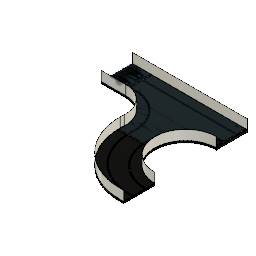
_1-5 (Entrance).d2b125fc-16cf-42d4-bfd9-f85618610363 (Autodesk Fusion 360 design; units mm, degrees)
Autodesk Fusion 360 part; units mm, degrees
note: some values were not read from the file. Chosen so that the rebuilt part matches the saved one: which bodies a step acts on. Set by a fixed rule: which sketch regions a step uses.
sketch "Sketch1" plane through (0, 0, 0) normal (0, 0, 1) x (1, 0, 0)
  line L0 (0, 0) -> (609.6, 0)
  line L1 (609.6, -812.8) -> (0, -812.8)
  line L2 (0, -812.8) -> (0, 0)
  line L3 (0, 0) -> (3022.6, 0)
  line L4 (3022.6, 0) -> (0, 0)
  line L5 (0, 0) -> (0, -812.8)
  line L6 (0, -812.8) -> (3022.6, -812.8)
  line L7 (0, 0) -> (1320.8, 0)
  circle A0 centre (4656.6619, -4772.6092) radius 793.75
  circle A1 centre (4656.6619, -4772.6092) radius 1625.6
  circle A2 centre (2997.2, -1612.9) radius 1612.9
  circle A3 centre (2997.2, -1612.9) radius 800.1
  line L8 (2997.2, -1612.9) -> (2997.2, 0)
  line L9 (2997.2, -1612.9) -> (2997.2, -3225.8)
  line L10 (3022.6, 0) -> (2997.2, 0)
  line L11 (2997.2, 0) -> (2997.2, -812.8)
  line L12 (2997.2, -812.8) -> (3022.6, -812.8)
  line L13 (2997.2, -1612.9) -> (1295.4, -1612.9)
  arc A4 (1384.3, -1612.9) -> (2997.2, -3225.8) centre (2997.2, -1612.9) ccw
  arc A5 (1384.3, -1612.9) -> (2997.2, -3225.8) centre (2997.2, -1612.9) ccw
  line L14 (2997.2, -1612.9) -> (1806.0752, -2792.535)
  arc A6 (1295.4, -1612.9) -> (2997.2, -3225.8) centre (2908.8371, -1614.7833) ccw
  arc A7 (2997.2, 0) -> (1295.4, -1612.9) centre (2908.8371, -1611.0167) ccw
  circle A8 centre (639.1793, -1473.2) radius 660.4
  dimension "d1" = 609.6
  dimension "d2" = 812.8
  dimension "d4" = 3022.6
  dimension "d8" = 1320.8
  dimension "d10" = 1587.5
  dimension "d11" = 3251.2
  dimension "d14" = 25.4
  dimension "d15" = 1701.8
  dimension "d16" = 1676.4
  dimension "d18" = 1320.8
  constraint horizontal L0
  constraint horizontal L1
  constraint vertical L2
  constraint coincident L0.start L2.end
  constraint perpendicular L2 L3
  constraint horizontal L4
  constraint vertical L5
  constraint horizontal L6
  constraint perpendicular L5 L7
  constraint concentric A0 A1
  constraint concentric A2 A3
  constraint coincident A2.centre A3.centre
  constraint coincident A2 L8.end
  constraint vertical L8
  constraint coincident A2 L9.end
  constraint parallel L8 L9
  constraint horizontal L10
  constraint vertical L11
  constraint horizontal L12
  constraint coincident L14.end A6
  constraint symmetric L9.end L13 L8.end
  constraint symmetric A6.start L13 A7.end
  constraint symmetric L13 A6 A7
  constraint tangent L6 A8
  constraint tangent A7 A8
  measures "d1" distance of L0.start L0.end
  measures "d2" distance of L0.start L1.end
  measures "d4" distance of L0.start L3.end
  measures "d8" distance of L0.start L7.end
  measures "d10" diameter of A0
  measures "d11" diameter of A1
  measures "d14" distance of L3.end L8.end
  measures "d15" distance of A2.centre L13.end
  measures "d16" distance of A2.centre L14.end
  measures "d18" diameter of A8
extrude "Extrude1" add sketch "Sketch1" along normal blind 50.8 contours L0 L1 L2 L3 L4 L5 L6 L7 A7 | L3 L4 L6 A2 A7 | L6 A7 A8 | L6 A2 L8 L11 | L6 A2 L13 A7 | L6 A2 A3 L13 | A2 L13 A4 A5 L14 A6 | A2 A4 A5 L14 A6 | A2 A3 L9 A4 A5 L14 | A2 A3 L13 A4 A5 L14 makes body 1
sketch "Lines" plane through (0, 0, 50.8) normal (0, 0, 1) x (-1, 0, 0)
  arc A0 (-1295.4, 1612.9) -> (-2997.2, 3225.8) centre (-2908.8371, 1614.7833) ccw
  line L0 (-2997.2, 3225.8) -> (-2997.2, 2413)
  arc A1 (-2997.2, 812.8) -> (-2997.2, 2413) centre (-2997.2, 1612.9) ccw
  line L1 (-2997.2, 812.8) -> (-2997.2, 0)
  line L2 (-2997.2, 0) -> (0, 0)
  line L3 (0, 0) -> (0, 812.8)
  line L4 (0, 812.8) -> (-639.1793, 812.8)
  arc A2 (-1298.3651, 1513.2267) -> (-639.1793, 812.8) centre (-639.1793, 1473.2) ccw
  arc A3 (-1298.3651, 1513.2267) -> (-1295.4, 1612.9) centre (-2908.8371, 1611.0167) ccw
  line L5 (0, 431.8) -> (-482.6, 431.8)
  line L6 (-482.6, 431.8) -> (-511.175, 431.8)
  line L7 (-511.175, 431.8) -> (-511.175, 812.8)
  line L8 (-511.175, 812.8) -> (-482.6, 812.8)
  line L9 (-482.6, 812.8) -> (-482.6, 431.8)
  line L10 (-511.175, 812.8) -> (-482.6, 812.8)
  line L11 (-482.6, 812.8) -> (-482.6, 0)
  line L12 (-482.6, 0) -> (-511.175, 0)
  line L13 (-511.175, 0) -> (-511.175, 812.8)
  line L14 (-1651, 0) -> (-1651, 1651)
  line L15 (-1651, 1651) -> (-1291.2162, 1651)
  line L16 (-1291.2162, 1651) -> (-1291.2162, 1679.575)
  line L17 (-1291.2162, 1679.575) -> (-1651, 1679.575)
  line L18 (-1651, 1679.575) -> (-1651, 1651)
  line L19 (-1291.2162, 1679.575) -> (-2198.0077, 1679.575)
  line L20 (-2198.0077, 1679.575) -> (-2198.0077, 1651)
  line L21 (-2198.0077, 1651) -> (-1291.2162, 1651)
  line L22 (-1291.2162, 1651) -> (-1291.2162, 1679.575)
  line L23 (0, 431.8) -> (-2946.4, 431.8)
  line L24 (-2946.4, 431.8) -> (-2974.975, 431.8)
  line L25 (-2974.975, 431.8) -> (-2974.975, 813.6871)
  line L26 (-2974.975, 813.6871) -> (-2946.4, 813.6871)
  line L27 (-2946.4, 813.6871) -> (-2946.4, 431.8)
  line L28 (-2974.975, 431.8) -> (-2946.4, 431.8)
  line L29 (-2946.4, 431.8) -> (-2946.4, 0)
  line L30 (-2946.4, 0) -> (-2974.975, 0)
  line L31 (-2974.975, 0) -> (-2974.975, 431.8)
  dimension "d45" = 482.6
  dimension "d46" = 28.575
  dimension "d47" = 1651
  dimension "d48" = 28.575
  dimension "d49" = 2946.4
  dimension "d50" = 28.575
  constraint coincident L3 L5.start
  constraint perpendicular L3 L5
  constraint horizontal L6
  constraint vertical L7
  constraint horizontal L8
  constraint vertical L9
  constraint horizontal L10
  constraint vertical L11
  constraint horizontal L12
  constraint vertical L13
  constraint coincident L2 L11.end
  constraint coincident L2 L14.start
  constraint perpendicular L2 L14
  constraint horizontal L15
  constraint vertical L16
  constraint horizontal L17
  constraint vertical L18
  constraint horizontal L19
  constraint vertical L20
  constraint horizontal L21
  constraint vertical L22
  constraint coincident A1 L20.end
  constraint perpendicular L11 L23
  constraint horizontal L24
  constraint vertical L25
  constraint horizontal L26
  constraint vertical L27
  constraint horizontal L28
  constraint vertical L29
  constraint horizontal L30
  constraint vertical L31
  constraint coincident L2 L29.end
  measures "d45" distance of L5.start L5.end
  measures "d46" distance of L5.end L6.end
  measures "d47" distance of L14.start L14.end
  measures "d48" distance of L14.end L17.end
  measures "d49" distance of L5.start L23.end
  measures "d50" distance of L23.end L24.end
extrude "Extrude6" add sketch "Lines" along normal blind 0.0254 contours A0 L15 L17 L18 L19 L21 | L18 L19 L20 L21 | L4 L6 L7 L8 L9 L10 L11 L13 L23 | L2 L6 L11 L12 L13 L23 | L2 L24 L28 L29 L30 L31 | A1 L24 L25 L26 L27 L28 bodies 1
sketch "Sketch7" plane through (0, 0, 50.8) normal (0, 0, 1) x (-1, 0, 0)
  line L0 (-2959.5333, 813.6871) -> (-2946.4, 813.6871)
  line L1 (-2946.4, 813.6871) -> (-2946.4, 0)
  line L2 (-2946.4, 0) -> (-511.175, 0)
  line L3 (-511.175, 0) -> (-511.175, 812.8)
  line L4 (-511.175, 812.8) -> (-639.1793, 812.8)
  arc A0 (-1298.3651, 1513.2267) -> (-639.1793, 812.8) centre (-639.1793, 1473.2) ccw
  arc A1 (-1298.3651, 1513.2267) -> (-1295.4, 1612.9) centre (-2908.8371, 1611.0167) ccw
  arc A2 (-1295.4, 1612.9) -> (-1295.8054, 1651) centre (-2908.8371, 1614.7833) ccw
  line L5 (-1295.8054, 1651) -> (-2198.0077, 1651)
  arc A3 (-2959.5333, 813.6871) -> (-2198.0077, 1651) centre (-2997.2, 1612.9) ccw
  line L6 (-482.6, 812.8) -> (-482.6, 0)
  line L7 (-482.6, 0) -> (0, 0)
  line L8 (0, 0) -> (0, 812.8)
  line L9 (0, 812.8) -> (-482.6, 812.8)
  line L10 (-2198.0077, 1679.575) -> (-1296.7004, 1679.575)
  arc A4 (-1296.7004, 1679.575) -> (-2997.2, 3225.8) centre (-2908.8371, 1614.7833) ccw
  line L11 (-2997.2, 3225.8) -> (-2997.2, 2413)
  arc A5 (-2198.0077, 1651) -> (-2997.2, 2413) centre (-2997.2, 1612.9) ccw
  line L12 (-2198.0077, 1651) -> (-2198.0077, 1679.575)
  line L13 (-2997.2, 812.8) -> (-2997.2, 0)
  line L14 (-574.675, 749.3) -> (-639.1793, 749.3)
  arc A6 (-1361.7484, 1517.0754) -> (-639.1793, 749.3) centre (-639.1793, 1473.2) ccw
  arc A7 (-1361.7484, 1517.0754) -> (-1359.0773, 1587.5) centre (-2908.8371, 1611.0167) ccw
  line L15 (-1359.0773, 1587.5) -> (-2133.9736, 1587.5)
  arc A8 (-2882.9, 756.8974) -> (-2133.9736, 1587.5) centre (-2997.2, 1612.9) ccw
  line L16 (-2882.9, 756.8974) -> (-2882.9, 63.5)
  line L17 (-2882.9, 63.5) -> (-574.675, 63.5)
  line L18 (-574.675, 63.5) -> (-574.675, 749.3)
  circle A9 centre (-793.75, 765.9949) radius 16
  circle A10 centre (-2171.7977, 1358.9) radius 16
  circle A11 centre (-1353.9986, 1358.9) radius 16
  circle A12 centre (-2768.6, 63.5) radius 16
  dimension "d53" = 63.5
  dimension "d55" = 32
  dimension "d59" = 32
  dimension "d60" = 32
  dimension "d62" = 32
  measures "d55" diameter of A9
  measures "d59" diameter of A10
  measures "d60" diameter of A11
  measures "d62" diameter of A12
extrude "Extrude7" add sketch "Sketch7" along normal blind 0.0254 contours A6 A9 | A6 A9 | L17 A12 | L17 A12 | A6 A11 | A6 A11 | A8 A10 | A8 A10 bodies 1
sketch "Sketch8" plane through (0, 0, 50.8) normal (0, 0, 1) x (-1, 0, 0)
  line L0 (-482.6, 812.8) -> (-482.6, 0)
  line L1 (-482.6, 0) -> (0, 0)
  line L2 (0, 0) -> (0, 812.8)
  line L3 (0, 812.8) -> (-482.6, 812.8)
  line L4 (-482.6, 231.775) -> (0, 231.775)
  line L5 (-482.6, 250.825) -> (0, 250.825)
  line L6 (0, 561.975) -> (-482.6, 561.975)
  line L7 (0, 581.025) -> (-482.6, 581.025)
  dimension "d66" = -250.825
extrude "Extrude8" add sketch "Sketch8" along normal blind 0.0254 contours L0 L2 L6 L7 | L0 L2 L4 L5 bodies 1
sketch "Sketch9" plane through (0, 0, 50.8254) normal (0, 0, 1) x (-1, 0, 0)
  line L0 (-511.175, 0) -> (-482.6, 0)
  line L1 (-482.6, 0) -> (-482.6, 231.775)
  line L2 (-482.6, 231.775) -> (0, 231.775)
  line L3 (0, 231.775) -> (0, 250.825)
  line L4 (0, 250.825) -> (-482.6, 250.825)
  line L5 (-482.6, 250.825) -> (-482.6, 561.975)
  line L6 (-482.6, 561.975) -> (0, 561.975)
  line L7 (0, 561.975) -> (0, 581.025)
  line L8 (0, 581.025) -> (-482.6, 581.025)
  line L9 (-482.6, 581.025) -> (-482.6, 812.8)
  line L10 (-482.6, 812.8) -> (-511.175, 812.8)
  line L11 (-511.175, 812.8) -> (-511.175, 0)
  line L12 (-482.6, 231.775) -> (-482.5746, 231.775)
  line L13 (-482.5746, 231.775) -> (-482.5746, 250.825)
  line L14 (-482.5746, 250.825) -> (-482.6, 250.825)
  line L15 (-482.6, 250.825) -> (-482.6, 231.775)
  dimension "d71" = 0.0254
  constraint horizontal L12
  constraint vertical L13
  constraint horizontal L14
  constraint vertical L15
  constraint coincident L1.end L2.start
  measures "d71" distance of L1.end L12.end
extrude "Extrude9" cut sketch "Sketch9" against normal blind 0.0254 contours L2 L4 L12 L13 L14 L15 bodies 1
sketch "Sketch10" plane through (0, 0, 50.8) normal (0, 0, 1) x (-1, 0, 0)
  line L0 (-482.6, 581.025) -> (0, 581.025)
  line L1 (0, 581.025) -> (0, 812.8)
  line L2 (0, 812.8) -> (-482.6, 812.8)
  line L3 (-482.6, 812.8) -> (-482.6, 581.025)
sketch "Sketch11" plane through (0, 0, 50.8254) normal (0, 0, 1) x (-1, 0, 0)
  line L0 (-482.6, 0) -> (-482.6, 561.975)
  line L1 (-482.6, 561.975) -> (0, 561.975)
  line L2 (0, 561.975) -> (0, 581.025)
  line L3 (0, 581.025) -> (-482.6, 581.025)
  line L4 (-482.6, 581.025) -> (-482.6, 812.8)
  line L5 (-482.6, 812.8) -> (-511.175, 812.8)
  line L6 (-511.175, 812.8) -> (-511.175, 0)
  line L7 (-511.175, 0) -> (-482.6, 0)
  line L8 (-482.6, 561.975) -> (-482.5746, 561.975)
  line L9 (-482.5746, 561.975) -> (-482.5746, 581.025)
  line L10 (-482.5746, 581.025) -> (-482.6, 581.025)
  line L11 (-482.6, 581.025) -> (-482.6, 561.975)
  dimension "d74" = 0.0254
  constraint horizontal L8
  constraint vertical L9
  constraint horizontal L10
  constraint vertical L11
  constraint coincident L0.end L1.start
  measures "d74" distance of L0.end L8.end
extrude "Extrude10" cut sketch "Sketch11" against normal blind 0.0254 contours L1 L3 L8 L9 L10 L11 bodies 1
sketch "Sketch12" plane through (0, 0, 50.8) normal (0, 0, 1) x (-1, 0, 0)
  circle A0 centre (-2768.6, 63.5) radius 16
  circle A1 centre (-793.75, 765.9949) radius 16
  circle A2 centre (-2171.7977, 1358.9) radius 16
  circle A3 centre (-1353.9986, 1358.9) radius 16
  line L0 (-2959.5333, 813.6871) -> (-2946.4, 813.6871)
  line L1 (-2946.4, 813.6871) -> (-2946.4, 0)
  line L2 (-2946.4, 0) -> (-511.175, 0)
  line L3 (-511.175, 0) -> (-511.175, 812.8)
  line L4 (-511.175, 812.8) -> (-639.1793, 812.8)
  arc A4 (-1298.3651, 1513.2267) -> (-639.1793, 812.8) centre (-639.1793, 1473.2) ccw
  arc A5 (-1298.3651, 1513.2267) -> (-1295.4, 1612.9) centre (-2908.8371, 1611.0167) ccw
  arc A6 (-1295.4, 1612.9) -> (-1295.8054, 1651) centre (-2908.8371, 1614.7833) ccw
  line L5 (-1295.8054, 1651) -> (-2198.0077, 1651)
  arc A7 (-2959.5333, 813.6871) -> (-2198.0077, 1651) centre (-2997.2, 1612.9) ccw
  line L6 (-2946.4, 250.825) -> (-511.175, 250.825)
  line L7 (-2946.4, 231.775) -> (-511.175, 231.775)
  dimension "d78" = -231.775
extrude "Extrude11" add sketch "Sketch12" along normal blind 0.0254 contours L1 L3 L6 L7 bodies 1
sketch "Sketch13" plane through (0, 0, 50.8254) normal (0, 0, 1) x (-1, 0, 0)
  line L0 (-482.6, 0) -> (-482.6, 812.8)
  line L1 (-482.6, 812.8) -> (-511.175, 812.8)
  line L2 (-511.175, 812.8) -> (-511.175, 250.825)
  line L3 (-511.175, 250.825) -> (-2946.4, 250.825)
  line L4 (-2946.4, 250.825) -> (-2946.4, 813.6871)
  line L5 (-2946.4, 813.6871) -> (-2959.5333, 813.6871)
  arc A0 (-2974.975, 813.1087) -> (-2959.5333, 813.6871) centre (-2997.2, 1612.9) ccw
  line L6 (-2974.975, 813.1087) -> (-2974.975, 0)
  line L7 (-2974.975, 0) -> (-2946.4, 0)
  line L8 (-2946.4, 0) -> (-2946.4, 231.775)
  line L9 (-2946.4, 231.775) -> (-511.175, 231.775)
  line L10 (-511.175, 231.775) -> (-511.175, 0)
  line L11 (-511.175, 0) -> (-482.6, 0)
  line L12 (-511.175, 250.825) -> (-511.2004, 250.825)
  line L13 (-511.2004, 250.825) -> (-511.2004, 231.775)
  line L14 (-511.2004, 231.775) -> (-511.175, 231.775)
  line L15 (-511.175, 231.775) -> (-511.175, 250.825)
  dimension "d81" = 0.0254
  constraint horizontal L12
  constraint vertical L13
  constraint horizontal L14
  constraint vertical L15
  constraint coincident L2.end L3.start
  measures "d81" distance of L2.end L12.end
extrude "Extrude12" cut sketch "Sketch13" against normal blind 0.0254 contours L3 L9 L12 L13 L14 L15 bodies 1
sketch "Sketch14" plane through (0, 0, 50.8254) normal (0, 0, 1) x (-1, 0, 0)
  line L0 (-511.2004, 231.775) -> (-511.2004, 250.825)
  line L1 (-511.2004, 250.825) -> (-2946.4, 250.825)
  line L2 (-2946.4, 250.825) -> (-2946.4, 813.6871)
  line L3 (-2946.4, 813.6871) -> (-2959.5333, 813.6871)
  arc A0 (-2974.975, 813.1087) -> (-2959.5333, 813.6871) centre (-2997.2, 1612.9) ccw
  line L4 (-2974.975, 813.1087) -> (-2974.975, 0)
  line L5 (-2974.975, 0) -> (-2946.4, 0)
  line L6 (-2946.4, 0) -> (-2946.4, 231.775)
  line L7 (-2946.4, 231.775) -> (-511.2004, 231.775)
  line L8 (-2946.4, 250.825) -> (-2946.3746, 250.825)
  line L9 (-2946.3746, 250.825) -> (-2946.3746, 231.775)
  line L10 (-2946.3746, 231.775) -> (-2946.4, 231.775)
  line L11 (-2946.4, 231.775) -> (-2946.4, 250.825)
  dimension "d84" = 0.0254
  constraint horizontal L8
  constraint vertical L9
  constraint horizontal L10
  constraint vertical L11
  constraint coincident L1.end L2.start
  measures "d84" distance of L1.end L8.end
extrude "Extrude13" cut sketch "Sketch14" against normal blind 0.0254 contours L1 L7 L8 L9 L10 L11 bodies 1
sketch "Sketch15" plane through (0, 0, 50.8) normal (0, 0, 1) x (-1, 0, 0)
  line L0 (-2974.975, 0) -> (-2974.975, 813.1087)
  arc A0 (-2997.2, 812.8) -> (-2974.975, 813.1087) centre (-2997.2, 1612.9) ccw
  line L1 (-2997.2, 812.8) -> (-2997.2, 0)
  line L2 (-2997.2, 0) -> (-2974.975, 0)
  line L3 (-2997.2, 231.775) -> (-2974.975, 231.775)
  line L4 (-2997.2, 250.825) -> (-2974.975, 250.825)
extrude "Extrude14" add sketch "Sketch15" along normal blind 0.0254 contours L0 L1 L3 L4 bodies 1
sketch "Sketch16" plane through (0, 0, 50.8254) normal (0, 0, 1) x (-1, 0, 0)
  line L0 (-2946.4, 0) -> (-2946.4, 813.6871)
  line L1 (-2946.4, 813.6871) -> (-2959.5333, 813.6871)
  arc A0 (-2974.975, 813.1087) -> (-2959.5333, 813.6871) centre (-2997.2, 1612.9) ccw
  line L2 (-2974.975, 813.1087) -> (-2974.975, 250.825)
  line L3 (-2974.975, 250.825) -> (-2997.2, 250.825)
  line L4 (-2997.2, 250.825) -> (-2997.2, 231.775)
  line L5 (-2997.2, 231.775) -> (-2974.975, 231.775)
  line L6 (-2974.975, 231.775) -> (-2974.975, 0)
  line L7 (-2974.975, 0) -> (-2946.4, 0)
  line L8 (-2974.975, 231.775) -> (-2975.0004, 231.775)
  line L9 (-2975.0004, 231.775) -> (-2975.0004, 250.825)
  line L10 (-2975.0004, 250.825) -> (-2974.975, 250.825)
  line L11 (-2974.975, 250.825) -> (-2974.975, 231.775)
  dimension "d93" = 0.0254
  constraint horizontal L8
  constraint vertical L9
  constraint horizontal L10
  constraint vertical L11
  constraint coincident L5.end L6.start
  measures "d93" distance of L5.end L8.end
extrude "Extrude15" cut sketch "Sketch16" against normal blind 0.0254 contours L3 L5 L8 L9 L10 L11 bodies 1
sketch "Sketch17" plane through (0, 0, 50.8) normal (0, 0, 1) x (-1, 0, 0)
  line L0 (-2975.0004, 231.775) -> (-2997.2, 231.775)
  line L1 (-2997.2, 231.775) -> (-2997.2, 0)
  line L2 (-2997.2, 0) -> (-2974.975, 0)
  line L3 (-2974.975, 0) -> (-2974.975, 813.1087)
  arc A0 (-2997.2, 812.8) -> (-2974.975, 813.1087) centre (-2997.2, 1612.9) ccw
  line L4 (-2997.2, 812.8) -> (-2997.2, 250.825)
  line L5 (-2997.2, 250.825) -> (-2975.0004, 250.825)
  line L6 (-2975.0004, 250.825) -> (-2975.0004, 231.775)
sketch "Sketch18" plane through (0, 0, 50.8) normal (0, 0, 1) x (-1, 0, 0)
  line L0 (-2946.3746, 250.825) -> (-511.2004, 250.825)
  line L1 (-511.2004, 250.825) -> (-511.2004, 231.775)
  line L2 (-511.2004, 231.775) -> (-2946.3746, 231.775)
  line L3 (-2946.3746, 231.775) -> (-2946.3746, 250.825)
  circle A0 centre (-2768.6, 63.5) radius 16
  line L4 (-2946.4, 813.6871) -> (-2946.4, 0)
  line L5 (-2946.4, 0) -> (-511.175, 0)
  line L6 (-511.175, 0) -> (-511.175, 812.8)
  line L7 (-511.175, 812.8) -> (-639.1793, 812.8)
  arc A1 (-1298.3651, 1513.2267) -> (-639.1793, 812.8) centre (-639.1793, 1473.2) ccw
  arc A2 (-1298.3651, 1513.2267) -> (-1295.4, 1612.9) centre (-2908.8371, 1611.0167) ccw
  arc A3 (-1295.4, 1612.9) -> (-1295.8054, 1651) centre (-2908.8371, 1614.7833) ccw
  line L8 (-1295.8054, 1651) -> (-2198.0077, 1651)
  arc A4 (-2959.5333, 813.6871) -> (-2198.0077, 1651) centre (-2997.2, 1612.9) ccw
  line L9 (-2959.5333, 813.6871) -> (-2946.4, 813.6871)
  circle A5 centre (-793.75, 765.9949) radius 16
  circle A6 centre (-2171.7977, 1358.9) radius 16
  circle A7 centre (-1353.9986, 1358.9) radius 16
  arc A8 (-1548.729, 1528.4291) -> (-639.1793, 561.975) centre (-639.1793, 1473.2) ccw
  line L10 (-511.175, 561.975) -> (-639.1793, 561.975)
  arc A9 (-1529.714, 1527.2745) -> (-639.1793, 581.025) centre (-639.1793, 1473.2) ccw
  line L11 (-511.175, 581.025) -> (-639.1793, 581.025)
  arc A10 (-1529.714, 1527.2745) -> (-1527.1752, 1612.9) centre (-2908.8371, 1611.0167) ccw
  arc A11 (-1527.1752, 1612.9) -> (-1527.522, 1645.7974) centre (-2908.8371, 1614.7833) ccw
  arc A12 (-1548.729, 1528.4291) -> (-1546.2252, 1612.9) centre (-2908.8371, 1611.0167) ccw
  arc A13 (-1546.2252, 1612.9) -> (-1546.5672, 1645.3698) centre (-2908.8371, 1614.7833) ccw
  line L12 (-1527.522, 1645.7974) -> (-1527.522, 1651)
  line L13 (-1546.5672, 1645.3698) -> (-1546.5672, 1651)
  line L14 (-1527.522, 1651) -> (-1546.5672, 1651)
  dimension "d96" = -250.825
  dimension "d97" = -231.775
  dimension "d99" = -250.825
  constraint vertical L12
  constraint coincident L8 L12.end
  constraint vertical L13
  constraint coincident L8 L13.end
extrude "Extrude16" add sketch "Sketch18" along normal blind 0.0254 contours L6 L8 A8 L10 A9 L11 A10 A11 A12 A13 L12 L13 L14 bodies 1
sketch "Sketch19" plane through (0, 0, 50.8254) normal (0, 0, 1) x (-1, 0, 0)
  line L0 (-2198.0077, 1651) -> (-1546.5672, 1651)
  line L1 (-1546.5672, 1651) -> (-1546.5672, 1645.3698)
  arc A0 (-1546.2252, 1612.9) -> (-1546.5672, 1645.3698) centre (-2908.8371, 1614.7833) ccw
  arc A1 (-1548.729, 1528.4291) -> (-1546.2252, 1612.9) centre (-2908.8371, 1611.0167) ccw
  arc A2 (-1548.729, 1528.4291) -> (-639.1793, 561.975) centre (-639.1793, 1473.2) ccw
  line L2 (-639.1793, 561.975) -> (-511.175, 561.975)
  line L3 (-511.175, 561.975) -> (-511.175, 0)
  line L4 (-511.175, 0) -> (-482.6, 0)
  line L5 (-482.6, 0) -> (-482.6, 812.8)
  line L6 (-482.6, 812.8) -> (-511.175, 812.8)
  line L7 (-511.175, 812.8) -> (-511.175, 581.025)
  line L8 (-511.175, 581.025) -> (-639.1793, 581.025)
  arc A3 (-1529.714, 1527.2745) -> (-639.1793, 581.025) centre (-639.1793, 1473.2) ccw
  arc A4 (-1529.714, 1527.2745) -> (-1527.1752, 1612.9) centre (-2908.8371, 1611.0167) ccw
  arc A5 (-1527.1752, 1612.9) -> (-1527.522, 1645.7974) centre (-2908.8371, 1614.7833) ccw
  line L9 (-1527.522, 1645.7974) -> (-1527.522, 1651)
  line L10 (-1527.522, 1651) -> (-1295.8054, 1651)
  arc A6 (-1295.8054, 1651) -> (-1296.7004, 1679.575) centre (-2908.8371, 1614.7833) ccw
  line L11 (-1296.7004, 1679.575) -> (-2198.0077, 1679.575)
  line L12 (-2198.0077, 1679.575) -> (-2198.0077, 1651)
  line L13 (-511.175, 561.975) -> (-511.2004, 561.975)
  line L14 (-511.2004, 561.975) -> (-511.2004, 581.025)
  line L15 (-511.2004, 581.025) -> (-511.175, 581.025)
  line L16 (-511.175, 581.025) -> (-511.175, 561.975)
  dimension "d102" = 0.0254
  constraint horizontal L13
  constraint vertical L14
  constraint horizontal L15
  constraint vertical L16
  constraint coincident L2.end L3.start
  measures "d102" distance of L2.end L13.end
extrude "Extrude17" cut sketch "Sketch19" against normal blind 0.0254 contours L2 L8 L13 L14 L15 L16 bodies 1
sketch "Sketch20" plane through (0, 0, 50.8254) normal (0, 0, 1) x (-1, 0, 0)
  line L0 (-511.2004, 561.975) -> (-511.2004, 581.025)
  line L1 (-511.2004, 581.025) -> (-639.1793, 581.025)
  arc A0 (-1529.714, 1527.2745) -> (-639.1793, 581.025) centre (-639.1793, 1473.2) ccw
  arc A1 (-1529.714, 1527.2745) -> (-1527.1752, 1612.9) centre (-2908.8371, 1611.0167) ccw
  arc A2 (-1527.1752, 1612.9) -> (-1527.522, 1645.7974) centre (-2908.8371, 1614.7833) ccw
  line L2 (-1527.522, 1645.7974) -> (-1527.522, 1651)
  line L3 (-1527.522, 1651) -> (-1295.8054, 1651)
  arc A3 (-1295.8054, 1651) -> (-1296.7004, 1679.575) centre (-2908.8371, 1614.7833) ccw
  line L4 (-1296.7004, 1679.575) -> (-2198.0077, 1679.575)
  line L5 (-2198.0077, 1679.575) -> (-2198.0077, 1651)
  line L6 (-2198.0077, 1651) -> (-1546.5672, 1651)
  line L7 (-1546.5672, 1651) -> (-1546.5672, 1645.3698)
  arc A4 (-1546.2252, 1612.9) -> (-1546.5672, 1645.3698) centre (-2908.8371, 1614.7833) ccw
  arc A5 (-1548.729, 1528.4291) -> (-1546.2252, 1612.9) centre (-2908.8371, 1611.0167) ccw
  arc A6 (-1548.729, 1528.4291) -> (-639.1793, 561.975) centre (-639.1793, 1473.2) ccw
  line L8 (-639.1793, 561.975) -> (-511.2004, 561.975)
  line L9 (-1527.522, 1651) -> (-1546.5672, 1651)
  line L10 (-1546.5672, 1651) -> (-1546.5672, 1650.9746)
  line L11 (-1546.5672, 1650.9746) -> (-1527.522, 1650.9746)
  line L12 (-1527.522, 1650.9746) -> (-1527.522, 1651)
  dimension "d105" = 0.0254
  constraint horizontal L9
  constraint vertical L10
  constraint horizontal L11
  constraint vertical L12
  constraint coincident L2.end L3.start
  measures "d105" distance of L2.end L11.end
extrude "Extrude18" cut sketch "Sketch20" against normal blind 0.0254 contours L2 L7 L9 L10 L11 L12 bodies 1
sketch "Sketch21" plane through (0, 0, 50.8) normal (0, 0, 1) x (-1, 0, 0)
  line L0 (-1527.522, 1650.9746) -> (-1527.522, 1645.7974)
  arc A0 (-1527.1752, 1612.9) -> (-1527.522, 1645.7974) centre (-2908.8371, 1614.7833) ccw
  arc A1 (-1529.714, 1527.2745) -> (-1527.1752, 1612.9) centre (-2908.8371, 1611.0167) ccw
  arc A2 (-1529.714, 1527.2745) -> (-639.1793, 581.025) centre (-639.1793, 1473.2) ccw
  line L1 (-639.1793, 581.025) -> (-511.2004, 581.025)
  line L2 (-511.2004, 581.025) -> (-511.2004, 561.975)
  line L3 (-511.2004, 561.975) -> (-639.1793, 561.975)
  arc A3 (-1548.729, 1528.4291) -> (-639.1793, 561.975) centre (-639.1793, 1473.2) ccw
  arc A4 (-1548.729, 1528.4291) -> (-1546.2252, 1612.9) centre (-2908.8371, 1611.0167) ccw
  arc A5 (-1546.2252, 1612.9) -> (-1546.5672, 1645.3698) centre (-2908.8371, 1614.7833) ccw
  line L4 (-1546.5672, 1645.3698) -> (-1546.5672, 1650.9746)
  line L5 (-1546.5672, 1650.9746) -> (-1527.522, 1650.9746)
  circle A6 centre (-1353.9986, 1358.9) radius 16
  circle A7 centre (-793.75, 765.9949) radius 16
  line L6 (-1295.8054, 1651) -> (-2198.0077, 1651)
  arc A8 (-2959.5333, 813.6871) -> (-2198.0077, 1651) centre (-2997.2, 1612.9) ccw
  line L7 (-2959.5333, 813.6871) -> (-2946.4, 813.6871)
  line L8 (-2946.4, 813.6871) -> (-2946.4, 0)
  line L9 (-2946.4, 0) -> (-511.175, 0)
  line L10 (-511.175, 0) -> (-511.175, 812.8)
  line L11 (-511.175, 812.8) -> (-639.1793, 812.8)
  arc A9 (-1298.3651, 1513.2267) -> (-639.1793, 812.8) centre (-639.1793, 1473.2) ccw
  arc A10 (-1298.3651, 1513.2267) -> (-1295.4, 1612.9) centre (-2908.8371, 1611.0167) ccw
  arc A11 (-1295.4, 1612.9) -> (-1295.8054, 1651) centre (-2908.8371, 1614.7833) ccw
  line L12 (-2946.3746, 250.825) -> (-511.2004, 250.825)
  line L13 (-511.2004, 250.825) -> (-511.2004, 231.775)
  line L14 (-511.2004, 231.775) -> (-2946.3746, 231.775)
  line L15 (-2946.3746, 231.775) -> (-2946.3746, 250.825)
  circle A12 centre (-2768.6, 63.5) radius 16
  circle A13 centre (-2171.7977, 1358.9) radius 16
  arc A14 (-2947.7252, 563.1402) -> (-1947.4672, 1662.944) centre (-2997.2, 1612.9) ccw
  arc A15 (-2948.622, 582.1691) -> (-1966.4956, 1662.0369) centre (-2997.2, 1612.9) ccw
  dimension "d108" = 250.825
  dimension "d109" = 231.775
extrude "Extrude19" add sketch "Sketch21" along normal blind 0.0279 contours L6 L8 A14 A15 bodies 1
sketch "Sketch22" plane through (0, 0, 50.8) normal (0, 0, 1) x (-1, 0, 0)
sketch "Sketch23" plane through (0, 0, 50.8) normal (0, 0, 1) x (-1, 0, 0)
  line L0 (-1527.522, 1650.9746) -> (-1527.522, 1645.7974)
  arc A0 (-1527.1752, 1612.9) -> (-1527.522, 1645.7974) centre (-2908.8371, 1614.7833) ccw
  arc A1 (-1529.714, 1527.2745) -> (-1527.1752, 1612.9) centre (-2908.8371, 1611.0167) ccw
  arc A2 (-1529.714, 1527.2745) -> (-639.1793, 581.025) centre (-639.1793, 1473.2) ccw
  line L1 (-639.1793, 581.025) -> (-511.2004, 581.025)
  line L2 (-511.2004, 581.025) -> (-511.2004, 561.975)
  line L3 (-511.2004, 561.975) -> (-639.1793, 561.975)
  arc A3 (-1548.729, 1528.4291) -> (-639.1793, 561.975) centre (-639.1793, 1473.2) ccw
  arc A4 (-1548.729, 1528.4291) -> (-1546.2252, 1612.9) centre (-2908.8371, 1611.0167) ccw
  arc A5 (-1546.2252, 1612.9) -> (-1546.5672, 1645.3698) centre (-2908.8371, 1614.7833) ccw
  line L4 (-1546.5672, 1645.3698) -> (-1546.5672, 1650.9746)
  line L5 (-1546.5672, 1650.9746) -> (-1527.522, 1650.9746)
  circle A6 centre (-1353.9986, 1358.9) radius 16
  circle A7 centre (-793.75, 765.9949) radius 16
  arc A8 (-2946.4, 563.2035) -> (-1946.9659, 1651) centre (-2997.2, 1612.9) ccw
  line L6 (-2946.4, 563.2035) -> (-2946.4, 0)
  line L7 (-2946.4, 0) -> (-511.175, 0)
  line L8 (-511.175, 0) -> (-511.175, 812.8)
  line L9 (-511.175, 812.8) -> (-639.1793, 812.8)
  arc A9 (-1298.3651, 1513.2267) -> (-639.1793, 812.8) centre (-639.1793, 1473.2) ccw
  arc A10 (-1298.3651, 1513.2267) -> (-1295.4, 1612.9) centre (-2908.8371, 1611.0167) ccw
  arc A11 (-1295.4, 1612.9) -> (-1295.8054, 1651) centre (-2908.8371, 1614.7833) ccw
  line L10 (-1295.8054, 1651) -> (-1946.9659, 1651)
  line L11 (-2946.3746, 250.825) -> (-511.2004, 250.825)
  line L12 (-511.2004, 250.825) -> (-511.2004, 231.775)
  line L13 (-511.2004, 231.775) -> (-2946.3746, 231.775)
  line L14 (-2946.3746, 231.775) -> (-2946.3746, 250.825)
  circle A12 centre (-2768.6, 63.5) radius 16
sketch "Sketch24" plane through (0, 0, 50.8) normal (0, 0, 1) x (-1, 0, 0)
  line L0 (-2997.2, 812.8) -> (-2997.2, 581.025)
  line L1 (-2997.2, 812.8) -> (-2997.2, 561.975)
  line L2 (-2997.2, 561.975) -> (-2974.975, 561.975)
  line L3 (-2974.975, 561.975) -> (-2974.975, 581.025)
  line L4 (-2974.975, 581.025) -> (-2997.2, 581.025)
  line L5 (-2997.2, 581.025) -> (-2997.2, 561.975)
  line L6 (-2974.975, 0) -> (-2974.975, 813.1087)
  point P0 (-2997.2, 812.8)
  dimension "d112" = 231.775
  dimension "d113" = 250.825
  constraint coincident P0 L0.start
  constraint parallel L0 L1
  constraint horizontal L2
  constraint vertical L3
  constraint horizontal L4
  constraint vertical L5
  constraint coincident L3.end L6
  measures "d112" distance of P0 L0.end
  measures "d113" distance of P0 L1.end
extrude "Extrude20" add sketch "Sketch24" along normal blind 0.0279 bodies 1
extrude "Extrude21" cut sketch "Sketch24" along normal blind 0.0279 bodies 1
extrude "Extrude22" add sketch "Sketch24" along normal blind 0.0279 bodies 1
sketch "Sketch25" plane through (0, 0, 50.8) normal (0, 0, 1) x (-1, 0, 0)
  line L0 (-2198.0077, 1679.575) -> (-1296.7004, 1679.575)
  arc A0 (-1296.7004, 1679.575) -> (-2997.2, 3225.8) centre (-2908.8371, 1614.7833) ccw
  line L1 (-2997.2, 3225.8) -> (-2997.2, 2413)
  arc A1 (-2198.0077, 1651) -> (-2997.2, 2413) centre (-2997.2, 1612.9) ccw
  line L2 (-2198.0077, 1651) -> (-2198.0077, 1679.575)
  arc A2 (-1966.4956, 1662.0369) -> (-2997.2, 2644.775) centre (-2997.2, 1612.9) ccw
  arc A3 (-1947.4672, 1662.944) -> (-2997.2, 2663.825) centre (-2997.2, 1612.9) ccw
  dimension "d121" = 250.825
extrude "Extrude23" add sketch "Sketch25" along normal blind 0.0279 contours L0 L1 A2 A3 bodies 1
sketch "Sketch28" plane through (0, 0, 50.8) normal (0, 0, 1) x (-1, 0, 0)
  arc A0 (-1948.3922, 1679.575) -> (-2997.2, 2663.825) centre (-2997.2, 1612.9) ccw
  line L0 (-1948.3922, 1679.575) -> (-1296.7004, 1679.575)
  arc A1 (-1296.7004, 1679.575) -> (-2997.2, 3225.8) centre (-2908.8371, 1614.7833) ccw
  line L1 (-2997.2, 3225.8) -> (-2997.2, 2663.825)
  arc A2 (-1547.323, 1669.5025) -> (-2983.4631, 2975.3514) centre (-2908.8371, 1614.7833) ccw
  arc A3 (-1528.2884, 1670.2675) -> (-2984.5064, 2994.3729) centre (-2908.8371, 1614.7833) ccw
  line L2 (-2983.4631, 2975.3514) -> (-2997.2, 2974.598)
  line L3 (-2984.5064, 2994.3729) -> (-2997.2, 2993.6766)
  dimension "d125" = -231.775
  constraint coincident L1 L2.end
  constraint tangent A2 L2
  constraint coincident L1 L3.end
  constraint tangent A3 L3
extrude "Extrude24" add sketch "Sketch28" along normal blind 0.0279 contours L0 L1 A2 A3 L2 L3 bodies 1
sketch "Sketch29" plane through (0, 0, 0) normal (0, 0, -1) x (1, 0, 0)
  arc A0 (2997.2, 3225.8) -> (1295.4, 1612.9) centre (2908.8371, 1614.7833) ccw
  arc A1 (1295.4, 1612.9) -> (1298.3651, 1513.2267) centre (2908.8371, 1611.0167) ccw
  arc A2 (639.1793, 812.8) -> (1298.3651, 1513.2267) centre (639.1793, 1473.2) ccw
  line L0 (639.1793, 812.8) -> (0, 812.8)
  line L1 (0, 812.8) -> (0, 0)
  line L2 (0, 0) -> (2997.2, 0)
  line L3 (2997.2, 0) -> (2997.2, 812.8)
  arc A3 (2997.2, 2413) -> (2997.2, 812.8) centre (2997.2, 1612.9) ccw
  line L4 (2997.2, 2413) -> (2997.2, 3225.8)
  arc A4 (1295.654, 1612.9) -> (1298.6187, 1513.2421) centre (2908.8371, 1611.0167) ccw
  arc A5 (639.1793, 812.546) -> (1298.6187, 1513.2421) centre (639.1793, 1473.2) ccw
  line L5 (639.1793, 812.546) -> (0.254, 812.546)
  line L6 (0.254, 812.546) -> (0.254, 0.254)
  line L7 (0.254, 0.254) -> (2996.946, 0.254)
  line L8 (2996.946, 0.254) -> (2996.946, 812.546)
  arc A6 (2996.946, 2413.254) -> (2996.946, 812.546) centre (2997.2, 1612.9) ccw
  line L9 (2996.946, 2413.254) -> (2996.946, 3225.5595)
  arc A7 (2996.946, 3225.5595) -> (1295.654, 1612.9) centre (2908.8371, 1614.7833) ccw
  dimension "d128" = 0.254
extrude "Extrude25" add sketch "Sketch29" along normal blind 254 separate body contours  makes body 2
move_body "Move1" bodies 2 to x (1, 0, 0) y (0, 1, 0) z (0, 0, 1) at (0, 0, 304.8)
sketch "Sketch30" plane through (0, 0, 304.8) normal (0, 0, 1) x (-1, 0, 0)
  line L0 (-2996.946, 2413.254) -> (-2996.946, 3225.5595)
  arc A0 (-1295.654, 1612.9) -> (-2996.946, 3225.5595) centre (-2908.8371, 1614.7833) ccw
  arc A1 (-1298.6187, 1513.2421) -> (-1295.654, 1612.9) centre (-2908.8371, 1611.0167) ccw
  arc A2 (-1298.6187, 1513.2421) -> (-639.1793, 812.546) centre (-639.1793, 1473.2) ccw
  line L1 (-639.1793, 812.546) -> (-0.254, 812.546)
  line L2 (-0.254, 812.546) -> (-0.254, 0.254)
  line L3 (-0.254, 0.254) -> (-2996.946, 0.254)
  line L4 (-2996.946, 0.254) -> (-2996.946, 812.546)
  arc A3 (-2996.946, 812.546) -> (-2996.946, 2413.254) centre (-2997.2, 1612.9) ccw
  line L5 (0, 812.8) -> (-639.1793, 812.8)
  arc A4 (-1298.3651, 1513.2267) -> (-639.1793, 812.8) centre (-639.1793, 1473.2) ccw
  arc A5 (-1298.3651, 1513.2267) -> (-1295.4, 1612.9) centre (-2908.8371, 1611.0167) ccw
  arc A6 (-1295.4, 1612.9) -> (-2997.2, 3225.8) centre (-2908.8371, 1614.7833) ccw
  line L6 (-2997.2, 3225.8) -> (-2997.2, 2413)
  arc A7 (-2997.2, 812.8) -> (-2997.2, 2413) centre (-2997.2, 1612.9) ccw
  line L7 (-2997.2, 812.8) -> (-2997.2, 0)
  line L8 (-2997.2, 0) -> (0, 0)
  line L9 (0, 0) -> (0, 812.8)
  line L10 (-0.254, 812.546) -> (0, 812.546)
  line L11 (-0.254, 0.254) -> (0, 0.254)
  constraint coincident L1.end L2.start
  constraint coincident L9 L10.end
  constraint perpendicular L9 L10
  constraint coincident L2.end L3.start
  constraint coincident L9 L11.end
  constraint perpendicular L9 L11
extrude "Extrude26" cut sketch "Sketch30" against normal blind 254 contours L2 L9 L10 L11 bodies 1 2
sketch "Sketch31" plane through (0, 0, 304.8) normal (0, 0, 1) x (-1, 0, 0)
  line L0 (0, 0.254) -> (-2996.946, 0.254)
  line L1 (-2996.946, 0.254) -> (-2996.946, 812.546)
  arc A0 (-2996.946, 812.546) -> (-2996.946, 2413.254) centre (-2997.2, 1612.9) ccw
  line L2 (-2996.946, 2413.254) -> (-2996.946, 3225.5595)
  arc A1 (-1295.654, 1612.9) -> (-2996.946, 3225.5595) centre (-2908.8371, 1614.7833) ccw
  arc A2 (-1298.6187, 1513.2421) -> (-1295.654, 1612.9) centre (-2908.8371, 1611.0167) ccw
  arc A3 (-1298.6187, 1513.2421) -> (-639.1793, 812.546) centre (-639.1793, 1473.2) ccw
  line L3 (-639.1793, 812.546) -> (0, 812.546)
  line L4 (0, 812.546) -> (0, 812.8)
  line L5 (0, 812.8) -> (-639.1793, 812.8)
  arc A4 (-1298.3651, 1513.2267) -> (-639.1793, 812.8) centre (-639.1793, 1473.2) ccw
  arc A5 (-1298.3651, 1513.2267) -> (-1295.4, 1612.9) centre (-2908.8371, 1611.0167) ccw
  arc A6 (-1295.4, 1612.9) -> (-2997.2, 3225.8) centre (-2908.8371, 1614.7833) ccw
  line L6 (-2997.2, 3225.8) -> (-2997.2, 2413)
  arc A7 (-2997.2, 812.8) -> (-2997.2, 2413) centre (-2997.2, 1612.9) ccw
  line L7 (-2997.2, 812.8) -> (-2997.2, 0)
  line L8 (-2997.2, 0) -> (0, 0)
  line L9 (0, 0) -> (0, 0.254)
sketch "Sketch32" plane through (0, 0, 304.8) normal (0, 0, 1) x (-1, 0, 0)
  line L0 (-2997.2, 3225.8) -> (-2997.2, 2413)
  line L1 (-2996.946, 3225.5595) -> (-2997.2, 3225.5595)
  point P0 (-2996.946, 3225.5595)
  constraint coincident P0 L1.start
  constraint coincident L0 L1.end
  constraint perpendicular L0 L1
sketch "Sketch33" plane through (0, 0, 304.8) normal (0, 0, 1) x (-1, 0, 0)
  line L0 (0, 0.254) -> (-2996.946, 0.254)
  line L1 (-2996.946, 0.254) -> (-2996.946, 812.546)
  arc A0 (-2996.946, 812.546) -> (-2996.946, 2413.254) centre (-2997.2, 1612.9) ccw
  line L2 (-2996.946, 2413.254) -> (-2996.946, 3225.5595)
  arc A1 (-1295.654, 1612.9) -> (-2996.946, 3225.5595) centre (-2908.8371, 1614.7833) ccw
  arc A2 (-1298.6187, 1513.2421) -> (-1295.654, 1612.9) centre (-2908.8371, 1611.0167) ccw
  arc A3 (-1298.6187, 1513.2421) -> (-639.1793, 812.546) centre (-639.1793, 1473.2) ccw
  line L3 (-639.1793, 812.546) -> (0, 812.546)
  line L4 (0, 812.546) -> (0, 812.8)
  line L5 (0, 812.8) -> (-639.1793, 812.8)
  arc A4 (-1298.3651, 1513.2267) -> (-639.1793, 812.8) centre (-639.1793, 1473.2) ccw
  arc A5 (-1298.3651, 1513.2267) -> (-1295.4, 1612.9) centre (-2908.8371, 1611.0167) ccw
  arc A6 (-1295.4, 1612.9) -> (-2997.2, 3225.8) centre (-2908.8371, 1614.7833) ccw
  line L6 (-2997.2, 3225.8) -> (-2997.2, 2413)
  arc A7 (-2997.2, 812.8) -> (-2997.2, 2413) centre (-2997.2, 1612.9) ccw
  line L7 (-2997.2, 812.8) -> (-2997.2, 0)
  line L8 (-2997.2, 0) -> (0, 0)
  line L9 (0, 0) -> (0, 0.254)
  line L10 (-2996.946, 3225.5595) -> (-2997.2, 3225.5595)
  line L11 (-2996.946, 2413.254) -> (-2997.2, 2413.254)
  constraint coincident L2.end A1.end
  constraint perpendicular L2 L10
  constraint coincident A0.end L2.start
  constraint coincident L6 L11.end
  constraint tangent A0 L11
extrude "Extrude27" cut sketch "Sketch33" against normal blind 254 contours L2 L6 L10 L11 bodies 1 2 makes body 3 at (1951.3332, -2913.386, 135.4667)
sketch "Sketch34" plane through (0, 0, 304.8) normal (0, 0, 1) x (-1, 0, 0)
  line L0 (-2996.946, 2413.254) -> (-2997.2, 2413.254)
  line L1 (-2997.2, 2413.254) -> (-2997.2, 2413)
  arc A0 (-2997.2, 812.8) -> (-2997.2, 2413) centre (-2997.2, 1612.9) ccw
  line L2 (-2997.2, 812.8) -> (-2997.2, 0)
  line L3 (-2997.2, 0) -> (0, 0)
  line L4 (0, 0) -> (0, 0.254)
  line L5 (0, 0.254) -> (-2996.946, 0.254)
  line L6 (-2996.946, 0.254) -> (-2996.946, 812.546)
  arc A1 (-2996.946, 812.546) -> (-2996.946, 2413.254) centre (-2997.2, 1612.9) ccw
  line L7 (-2996.946, 812.546) -> (-2997.2, 812.546)
  line L8 (-2996.946, 0.254) -> (-2997.2, 0.254)
  constraint coincident L6.end A1.start
  constraint coincident L2 L7.end
  constraint tangent A1 L7
  constraint coincident L5.end L6.start
  constraint coincident L2 L8.end
  constraint perpendicular L2 L8
extrude "Extrude28" cut sketch "Sketch34" against normal blind 254 contours L2 L6 L7 L8 bodies 1 2 makes body 4 at (2917.2738, -816.5469, 220.1333)
sketch "Sketch35" plane through (0, 0, 50.8) normal (0, 0, 1) x (-1, 0, 0)
  line L0 (-1527.522, 1650.9746) -> (-1527.522, 1645.7974)
  arc A0 (-1527.1752, 1612.9) -> (-1527.522, 1645.7974) centre (-2908.8371, 1614.7833) ccw
  arc A1 (-1529.714, 1527.2745) -> (-1527.1752, 1612.9) centre (-2908.8371, 1611.0167) ccw
  arc A2 (-1529.714, 1527.2745) -> (-639.1793, 581.025) centre (-639.1793, 1473.2) ccw
  line L1 (-639.1793, 581.025) -> (-511.2004, 581.025)
  line L2 (-511.2004, 581.025) -> (-511.2004, 561.975)
  line L3 (-511.2004, 561.975) -> (-639.1793, 561.975)
  arc A3 (-1548.729, 1528.4291) -> (-639.1793, 561.975) centre (-639.1793, 1473.2) ccw
  arc A4 (-1548.729, 1528.4291) -> (-1546.2252, 1612.9) centre (-2908.8371, 1611.0167) ccw
  arc A5 (-1546.2252, 1612.9) -> (-1546.5672, 1645.3698) centre (-2908.8371, 1614.7833) ccw
  line L4 (-1546.5672, 1645.3698) -> (-1546.5672, 1650.9746)
  line L5 (-1546.5672, 1650.9746) -> (-1527.522, 1650.9746)
  circle A6 centre (-1353.9986, 1358.9) radius 16
  circle A7 centre (-793.75, 765.9949) radius 16
  arc A8 (-2946.4, 563.2035) -> (-1946.9659, 1651) centre (-2997.2, 1612.9) ccw
  line L6 (-2946.4, 563.2035) -> (-2946.4, 0)
  line L7 (-2946.4, 0) -> (-511.175, 0)
  line L8 (-511.175, 0) -> (-511.175, 812.8)
  line L9 (-511.175, 812.8) -> (-639.1793, 812.8)
  arc A9 (-1298.3651, 1513.2267) -> (-639.1793, 812.8) centre (-639.1793, 1473.2) ccw
  arc A10 (-1298.3651, 1513.2267) -> (-1295.4, 1612.9) centre (-2908.8371, 1611.0167) ccw
  arc A11 (-1295.4, 1612.9) -> (-1295.8054, 1651) centre (-2908.8371, 1614.7833) ccw
  line L10 (-1295.8054, 1651) -> (-1946.9659, 1651)
  line L11 (-2946.3746, 250.825) -> (-511.2004, 250.825)
  line L12 (-511.2004, 250.825) -> (-511.2004, 231.775)
  line L13 (-511.2004, 231.775) -> (-2946.3746, 231.775)
  line L14 (-2946.3746, 231.775) -> (-2946.3746, 250.825)
  circle A12 centre (-2768.6, 63.5) radius 16
sketch "Sketch36" plane through (0, 0, 50.8) normal (0, 0, 1) x (-1, 0, 0)
  line L0 (0, 0) -> (0, 812.8)
  line L1 (0, 812.8) -> (-482.6, 812.8)
  line L2 (-482.6, 812.8) -> (-482.6, 0)
  line L3 (-482.6, 0) -> (0, 0)
  line L4 (-0.254, 581.025) -> (-0.254, 561.975)
  line L5 (-0.254, 561.975) -> (-482.5746, 561.975)
  line L6 (-482.5746, 561.975) -> (-482.5746, 581.025)
  line L7 (-482.5746, 581.025) -> (-0.254, 581.025)
  line L8 (-0.254, 250.825) -> (-0.254, 231.775)
  line L9 (-0.254, 231.775) -> (-482.5746, 231.775)
  line L10 (-482.5746, 231.775) -> (-482.5746, 250.825)
  line L11 (-482.5746, 250.825) -> (-0.254, 250.825)
  line L12 (-0.254, 571.5) -> (-241.4143, 571.5)
  line L13 (-419.2143, 469.9) -> (-63.6143, 469.9)
  line L14 (-63.6143, 469.9) -> (-63.6143, 673.1)
  line L15 (-63.6143, 673.1) -> (-419.2143, 673.1)
  line L16 (-419.2143, 673.1) -> (-419.2143, 469.9)
  line L17 (-419.2143, 469.9) -> (-63.6143, 673.1) construction
  line L18 (-63.6143, 469.9) -> (-419.2143, 673.1) construction
  line L19 (-50.9143, 685.8) -> (-431.9143, 685.8)
  line L20 (-431.9143, 685.8) -> (-431.9143, 457.2)
  line L21 (-431.9143, 457.2) -> (-50.9143, 457.2)
  line L22 (-50.9143, 457.2) -> (-50.9143, 685.8)
  point P0 (-241.4143, 571.5)
  dimension "d140" = 241.1603
  dimension "d141" = 355.6
  dimension "d142" = 203.2
  dimension "d143" = 12.7
  constraint midpoint L4 L12.start
  constraint perpendicular L6 L12
  constraint horizontal L13
  constraint perpendicular L13 L14
  constraint parallel L13 L15
  constraint parallel L14 L16
  constraint coincident L17 P0
  constraint coincident L18 P0
  constraint coincident P0 L12.end
  measures "d140" distance of L12.start P0
  measures "d141" distance of L14.end L15.end
  measures "d142" distance of L13.end L14.end
extrude "Extrude29" add sketch "Sketch36" along normal blind 0.0279 contours L7 L14 L15 L16 L19 L20 L22 | L5 L13 L14 L16 L20 L21 L22 bodies 1
sketch "Sketch37" plane through (0, 0, 50.8) normal (0, 0, 1) x (-1, 0, 0)
  line L0 (-0.254, 250.825) -> (-0.254, 231.775)
  line L1 (-0.254, 231.775) -> (-482.5746, 231.775)
  line L2 (-482.5746, 231.775) -> (-482.5746, 250.825)
  line L3 (-482.5746, 250.825) -> (-0.254, 250.825)
  line L4 (-431.9143, 581.025) -> (-431.9143, 685.8)
  line L5 (-431.9143, 685.8) -> (-50.9143, 685.8)
  line L6 (-50.9143, 685.8) -> (-50.9143, 581.025)
  line L7 (-50.9143, 581.025) -> (-0.254, 581.025)
  line L8 (-0.254, 581.025) -> (-0.254, 561.975)
  line L9 (-0.254, 561.975) -> (-50.9143, 561.975)
  line L10 (-50.9143, 561.975) -> (-50.9143, 457.2)
  line L11 (-50.9143, 457.2) -> (-431.9143, 457.2)
  line L12 (-431.9143, 457.2) -> (-431.9143, 561.975)
  line L13 (-431.9143, 561.975) -> (-482.5746, 561.975)
  line L14 (-482.5746, 561.975) -> (-482.5746, 581.025)
  line L15 (-482.5746, 581.025) -> (-431.9143, 581.025)
  line L16 (0, 0) -> (0, 812.8)
  line L17 (0, 812.8) -> (-482.6, 812.8)
  line L18 (-482.6, 812.8) -> (-482.6, 0)
  line L19 (-482.6, 0) -> (0, 0)
  line L20 (-0.254, 241.3) -> (-241.4143, 241.3)
  line L21 (-419.2143, 139.7) -> (-63.6143, 139.7)
  line L22 (-63.6143, 139.7) -> (-63.6143, 342.9)
  line L23 (-63.6143, 342.9) -> (-419.2143, 342.9)
  line L24 (-419.2143, 342.9) -> (-419.2143, 139.7)
  line L25 (-419.2143, 139.7) -> (-63.6143, 342.9) construction
  line L26 (-63.6143, 139.7) -> (-419.2143, 342.9) construction
  line L27 (-50.9143, 355.6) -> (-431.9143, 355.6)
  line L28 (-431.9143, 355.6) -> (-431.9143, 127)
  line L29 (-431.9143, 127) -> (-50.9143, 127)
  line L30 (-50.9143, 127) -> (-50.9143, 355.6)
  point P0 (-241.4143, 241.3)
  dimension "d146" = 241.1603
  dimension "d147" = 355.6
  dimension "d148" = 203.2
  dimension "d149" = 12.7
  constraint midpoint L0 L20.start
  constraint perpendicular L2 L20
  constraint horizontal L21
  constraint perpendicular L21 L22
  constraint parallel L21 L23
  constraint parallel L22 L24
  constraint coincident L25 P0
  constraint coincident L26 P0
  constraint coincident P0 L20.end
  measures "d146" distance of L20.start P0
  measures "d147" distance of L22.end L23.end
  measures "d148" distance of L21.end L22.end
extrude "Extrude30" add sketch "Sketch37" along normal blind 0.0279 contours L3 L22 L23 L24 L27 L28 L30 | L1 L21 L22 L24 L28 L29 L30 bodies 1
sketch "Sketch38" plane through (0, 0, 50.8) normal (0, 0, 1) x (-1, 0, 0)
  line L0 (-431.9143, 250.825) -> (-431.9143, 355.6)
  line L1 (-431.9143, 355.6) -> (-50.9143, 355.6)
  line L2 (-50.9143, 355.6) -> (-50.9143, 250.825)
  line L3 (-50.9143, 250.825) -> (-0.254, 250.825)
  line L4 (-0.254, 250.825) -> (-0.254, 231.775)
  line L5 (-0.254, 231.775) -> (-50.9143, 231.775)
  line L6 (-50.9143, 231.775) -> (-50.9143, 127)
  line L7 (-50.9143, 127) -> (-431.9143, 127)
  line L8 (-431.9143, 127) -> (-431.9143, 231.775)
  line L9 (-431.9143, 231.775) -> (-482.5746, 231.775)
  line L10 (-482.5746, 231.775) -> (-482.5746, 250.825)
  line L11 (-482.5746, 250.825) -> (-431.9143, 250.825)
  line L12 (-431.9143, 581.025) -> (-431.9143, 685.8)
  line L13 (-431.9143, 685.8) -> (-50.9143, 685.8)
  line L14 (-50.9143, 685.8) -> (-50.9143, 581.025)
  line L15 (-50.9143, 581.025) -> (-0.254, 581.025)
  line L16 (-0.254, 581.025) -> (-0.254, 561.975)
  line L17 (-0.254, 561.975) -> (-50.9143, 561.975)
  line L18 (-50.9143, 561.975) -> (-50.9143, 457.2)
  line L19 (-50.9143, 457.2) -> (-431.9143, 457.2)
  line L20 (-431.9143, 457.2) -> (-431.9143, 561.975)
  line L21 (-431.9143, 561.975) -> (-482.5746, 561.975)
  line L22 (-482.5746, 561.975) -> (-482.5746, 581.025)
  line L23 (-482.5746, 581.025) -> (-431.9143, 581.025)
  line L24 (0, 0) -> (0, 812.8)
  line L25 (0, 812.8) -> (-482.6, 812.8)
  line L26 (-482.6, 812.8) -> (-482.6, 0)
  line L27 (-482.6, 0) -> (0, 0)
  line L28 (-0.254, 571.5) -> (-241.4143, 571.5)
  line L29 (-0.254, 241.3) -> (-241.4143, 241.3)
  dimension "d152" = 241.1603
  dimension "d153" = 241.1603
  constraint midpoint L16 L28.start
  constraint perpendicular L22 L28
  constraint midpoint L4 L29.start
  constraint perpendicular L10 L29
  measures "d152" distance of L28.start L28.end
  measures "d153" distance of L29.start L29.end
equation "d18 = ( 26 * 2 ) * 1 in"
equation "d140 = 18.989 in / 2"
equation "d146 = 18.989 in / 2"
equation "d152 = 18.989 in / 2"
equation "d153 = 18.989 in / 2"
